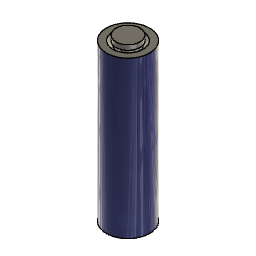
lithium ion battery (Autodesk Fusion 360 design; units mm, degrees)
Autodesk Fusion 360 part; units mm, degrees
note: some values were not read from the file. Chosen so that the rebuilt part matches the saved one: that a step has no effect.
sketch "Sketch1" plane through (0, 0, 0) normal (0, 0, 1) x (1, 0, 0)
  circle A0 centre (0, 0) radius 9
  dimension "d1" = 18
  constraint coincident A0.centre origin
  measures "d1" diameter of A0
extrude "Extrude1" add sketch "Sketch1" along normal blind 65 and the other way blind 0 makes body 1
hole "Hole1" at (0, 0, 65) direction (0, 0, -1) diameter 6.6 depth 60 tip angle 118 countersink diameter 12.6 countersink angle 90 bodies 1
sketch "Sketch2" plane through (0, 0, 0) normal (1, 0, 0) x (0, 1, 0)
sketch "Sketch3" plane through (0, 0, 0) normal (0, 0, 1) x (1, 0, 0)
  circle A0 centre (0, 0) radius 4.4213
  circle A1 centre (0, 0) radius 4.4213
  constraint coincident A0.centre A1.centre
  constraint concentric A0 A1
extrude "Extrude2" cut sketch "Sketch3" along normal blind 66 bodies 1
form "Form2" [no effect]
sketch "Sketch4" plane through (0, 0, 65) normal (0, 0, 1) x (-1, 0, 0)
  circle A0 centre (0, 0) radius 6.3
  circle A1 centre (0, 0) radius 9
  circle A2 centre (0, 0) radius 5
  dimension "d13" = 10
  constraint concentric A0 A2
  measures "d13" diameter of A2
extrude "Extrude3" add sketch "Sketch4" along normal blind 2 separate body contours A2 makes body 2
sketch "Sketch5" plane through (0, 0, 65) normal (0, 0, -1) x (1, 0, 0)
  circle A0 centre (0, 0) radius 5
  circle A1 centre (0, 0) radius 3
  dimension "d16" = 6
  constraint coincident A0.centre A1.centre
  measures "d16" diameter of A1
extrude "Extrude4" add sketch "Sketch5" along normal blind 65 contours A1 bodies 2
sketch "Sketch6" plane through (0, 0, 0) normal (0, 0, -1) x (1, 0, 0)
  circle A0 centre (0, 0) radius 3
form "Form3" [no effect]
